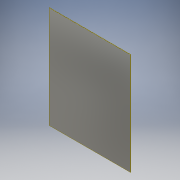
# Autodesk Inventor part: ReflectorWallWide
Saved by Autodesk Inventor 2017 (Build 210142000, 142)
## iProperties
Created: 2016-12-13
Part Number: ReflectorWallWide
Material: Silver
Document SubType Name: Modeling
Designer: umr
Density: 10.49 g/cm^3
Appearance: Silver
Author: umr
Autodesk Inventor part; units mm, degrees
ref_plane "YZ Plane" through (0, 0, 0) normal (1, 0, 0) x (0, 1, 0)
ref_plane "XZ Plane" through (0, 0, 0) normal (0, 1, 0) x (-1, 0, 0)
ref_plane "XY Plane" through (0, 0, 0) normal (0, 0, 1) x (1, 0, 0)
sketch "Sketch1" plane through (0, 0, 0) normal (0, 1, 0) x (-1, 0, 0)
  line L0 (0, 0) -> (1200, 0)
  line L1 (1200, 0) -> (1200, -1500)
  line L2 (1200, -1500) -> (0, -1500)
  line L3 (0, -1500) -> (0, 0)
  dimension "d0" = 1200
  dimension "d1" = 1500
  constraints: 8 end point, 2 parallel, 1 horizontal, 1 perpendicular
  measures "d0" distance of L1.end L2.end
  measures "d1" distance of L0.end L1.end
extrude "Extrusion1" add sketch "Sketch1" along normal blind 5
body "Solid1"
